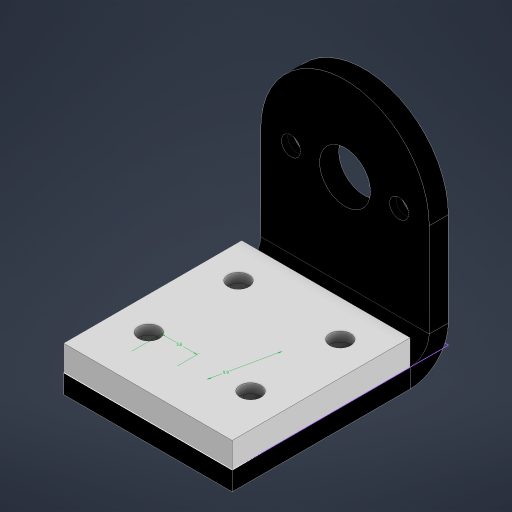
# Autodesk Inventor part: JGA25-370-bracket
Saved by Autodesk Inventor 2023 (Build 270158000, 158)
## iProperties
Created: 2022-05-10
Part Number: JGA25-370-bracket
Material: ABS Plastic
Document SubType Name: Sheet Metal
Designer: Dan
Density: 1.06 g/cm^3
Sheet Metal Rule: Default_mm
Appearance: Anodized - Black
Author: Dan
Autodesk Inventor part; units mm, degrees
ref_plane "YZ Plane" through (0, 0, 0) normal (1, 0, 0) x (0, 1, 0)
ref_plane "XZ Plane" through (0, 0, 0) normal (0, 1, 0) x (-1, 0, 0)
ref_plane "XY Plane" through (0, 0, 0) normal (0, 0, 1) x (1, 0, 0)
sketch "Sketch4" plane through (0, 0, 0) normal (0, 0, 1) x (1, 0, 0)
  line L0 (0, 0) -> (26.5, 0)
  line L1 (26.5, 0) -> (26.5, 20.75)
  line L2 (0, 20.75) -> (0, 0)
  arc A0 (26.5, 20.75) -> (0, 20.75) centre (13.25, 20.75) ccw
  line L3 (-1.1061, 34) -> (25.3939, 34) construction
  dimension "d70" = 26.5
  dimension "d71" = 34
  measures "d70" distance of L0.start L0.end
  measures "d71" distance between parallel lines of L3 L0
extrude "Plate3" add sketch "Sketch4" along normal blind 3
sketch "Sketch5" plane through (26.5, 3, 0) normal (0, -1, 0) x (1, 0, 0)
  line L0 (-26.5, 0) -> (0, 0)
  line L1 (0, 0) -> (0, 34)
  line L2 (0, 34) -> (-26.5, 34)
  line L3 (-26.5, 34) -> (-26.5, 0)
  constraints: 6 end point, 1 horizontal, 1 perpendicular, 1 vertical
edge flange "Flange2" height 34 angle 90 thickness 3 bend radius 3 thickness toward (0, -1, 0) relief tear relief width 3 relief depth 1.5 edges at (13.25, 0, 3) wall of the first edge with corners at (0, 3, 0) (26.5, 3, 0) (26.5, 3, 34) (0, 3, 34)
bend "Bend2"
corner "Corner2"
sketch "Sketch8" plane through (0, 3, 3) normal (0, 0, 1) x (1, 0, 0)
  line L0 (26.5, 3) -> (0, 3) projected
  line L1 (13.25, 3) -> (13.25, 35.5458) construction
  line L2 (0, -3) -> (26.5, -3) projected
  point P0 (13.25, 17.75)
  point P1 (13.25, -3)
  dimension "d72" = 20.75
  constraints: 2 end point, 2 midpoint, 1 point on line, 1 vertical
  measures "d72" distance of point (13.25, -3) point (13.25, 17.75)
hole "Hole3" at (13.25, 20.75, 3) direction (0, 0, -1) diameter 8 end through all
sketch "Sketch11" plane through (0, 3, 34) normal (0, 1, 0) x (1, 0, 0)
  line L0 (0, 0) -> (26.5, 0) projected
  line L1 (13.25, 0) -> (13.25, 41.3955) construction
  point P0 (0, 34)
  point P1 (13.25, 15.2)
  dimension "d81" = 15.2
  constraints: 2 end point, 1 midpoint, 1 point on line, 1 vertical
  measures "d81" distance from line of L0 point (13.25, 15.2)
hole "Hole5" at (13.25, 3, 18.8) direction (0, -1, 0) diameter 6.9 end through all
sketch "Sketch12" plane through (0, 3, 34) normal (0, 1, 0) x (1, 0, 0)
  circle A0 centre (13.25, 15.2) radius 3.45 projected
  circle A1 centre (13.25, 15.2) radius 10.6631 construction
  line L0 (0, 0) -> (26.5, 0) projected
  point P0 (0, 34)
  point P1 (21.25, 8.15)
  point P2 (5.25, 8.15)
  point P3 (5.25, 22.25)
  point P4 (21.25, 22.25)
  dimension "d89" = 16
  dimension "d90" = 8.15
  constraints: 4 point on circle, 2 horizontal alignment, 1 centre point, 1 coincident, 1 vertical alignment
  measures "d89" distance of point (5.25, 8.15) point (21.25, 8.15)
  measures "d90" distance from line of L0 point (21.25, 8.15)
hole "Hole6" at (21.25, 3, 25.85) at (5.25, 3, 25.85) at (5.25, 3, 11.75) at (21.25, 3, 11.75) direction (0, -1, 0) diameter 3.3 end through all
sketch "Sketch13" plane through (0, 0, 0) normal (0, 0, -1) x (-1, 0, 0)
  circle A0 centre (-13.25, 20.75) radius 4 projected
  circle A1 centre (-13.25, 20.75) radius 8.5 construction
  point P0 (0, 0)
  point P1 (-21.75, 20.75)
  point P2 (-4.75, 20.75)
  dimension "d98" = 17
  constraints: 2 horizontal alignment, 2 point on circle, 1 centre point, 1 coincident
  measures "d98" distance of A1.start A1.end
hole "Hole7" at (21.75, 20.75, 0) at (4.75, 20.75, 0) direction (0, 0, 1) diameter 3 end through all counterbore diameter 6 counterbore depth 2
sketch "Sketch14" plane through (0, 3, 34) normal (0, 1, 0) x (1, 0, 0)
  circle A0 centre (5.25, 8.15) radius 1.65 projected
  line L0 (2.45, 6.5334) -> (2.45, 9.7666)
  line L1 (2.45, 9.7666) -> (5.25, 11.3832)
  line L2 (5.25, 11.3832) -> (8.05, 9.7666)
  line L3 (8.05, 9.7666) -> (8.05, 6.5334)
  line L4 (8.05, 6.5334) -> (5.25, 4.9168)
  line L5 (5.25, 4.9168) -> (2.45, 6.5334)
  line L6 (0, 28) -> (0, 0) projected
  circle A1 centre (5.25, 22.25) radius 1.65 projected
  line L7 (2.45, 23.8666) -> (5.25, 25.4832)
  line L8 (5.25, 25.4832) -> (8.05, 23.8666)
  line L9 (8.05, 23.8666) -> (8.05, 20.6334)
  line L10 (8.05, 20.6334) -> (5.25, 19.0168)
  line L11 (5.25, 19.0168) -> (2.45, 20.6334)
  line L12 (2.45, 20.6334) -> (2.45, 23.8666)
  circle A2 centre (21.25, 8.15) radius 1.65 projected
  line L13 (18.45, 9.7666) -> (21.25, 11.3832)
  line L14 (21.25, 11.3832) -> (24.05, 9.7666)
  line L15 (24.05, 9.7666) -> (24.05, 6.5334)
  line L16 (24.05, 6.5334) -> (21.25, 4.9168)
  line L17 (21.25, 4.9168) -> (18.45, 6.5334)
  line L18 (18.45, 6.5334) -> (18.45, 9.7666)
  circle A3 centre (21.25, 22.25) radius 1.65 projected
  line L19 (18.45, 23.8666) -> (21.25, 25.4832)
  line L20 (21.25, 25.4832) -> (24.05, 23.8666)
  line L21 (24.05, 23.8666) -> (24.05, 20.6334)
  line L22 (24.05, 20.6334) -> (21.25, 19.0168)
  line L23 (21.25, 19.0168) -> (18.45, 20.6334)
  line L24 (18.45, 20.6334) -> (18.45, 23.8666)
  line L25 (26.5, 28) -> (26.5, 0) projected
  line L26 (0, 0) -> (26.5, 0) projected
  line L27 (26.5, 28) -> (0, 28)
  line L28 (0, 28) -> (0, 0)
  line L29 (0, 0) -> (26.5, 0)
  line L30 (26.5, 0) -> (26.5, 28)
  circle A4 centre (13.25, 15.2) radius 3.45 projected
  circle A5 centre (13.25, 15.2) radius 4.95
  point P0 (0, 34)
  point P1 (2.45, 8.15)
  point P2 (0, 28)
  dimension "d100" = 5.6
  dimension "d110" = 9.9
  constraints: 56 end point, 9 parallel, 6 coincident, 1 centre point, 1 horizontal, 1 midpoint, 1 perpendicular, 52 other
  measures "d100" distance from line of point (2.45, 8.15) L3
  measures "d110" diameter of A5
extrude "Extrusion1" add sketch "Sketch14" along normal blind 4 separate body contours A0 | L0 L1 L2 L3 L4 L5 | L27 L25 L26 L6 | A1 | L7 L8 L9 L10 L11 L12 | A2 | L13 L14 L15 L16 L17 L18 | A3 | L19 L20 L21 L22 L23 L24 | A4 | A5
extrude "Extrusion2" add sketch "Sketch14" against normal blind 2.5 contours A4 | A5 bodies 2
extrude "Extrusion3" cut sketch "Sketch14" along normal blind 2.5 contours A0 | L0 L1 L2 L3 L4 L5 | A1 | L7 L8 L9 L10 L11 L12 | A2 | L13 L14 L15 L16 L17 L18 | A3 | L19 L20 L21 L22 L23 L24 bodies 2
extrude "Extrusion4" cut sketch "Sketch14" along normal blind 9 contours A0 | A1 | A2 | A3 bodies 2
equation "\"d27\" = Thickness"
equation "\"d28\" = BendReliefWidth"
equation "\"d29\" = BendReliefDepth"
equation "\"d30\" = MinimumRemnant"
equation "\"d31\" = TransitionRadius"
equation "\"d34\" = BendRadius"
equation "\"d35\" = CornerReliefSize"
equation "\"d36\" = GapSize"
equation "\"d37\" = JacobiRadiusSize"
equation "\"BendRadius\" = Thickness"
equation "\"BendReliefWidth\" = Thickness"
equation "\"BendReliefDepth\" = 0.5 * Thickness"
equation "\"CornerReliefSize\" = 4 * Thickness"
equation "\"MinimumRemnant\" = 2 * Thickness"
equation "\"TransitionRadius\" = BendRadius"
equation "\"JacobiRadiusSize\" = BendRadius"
equation "\"GapSize\" = Thickness"
equation "\"Thickness\" = 3"
body "Solid2"
